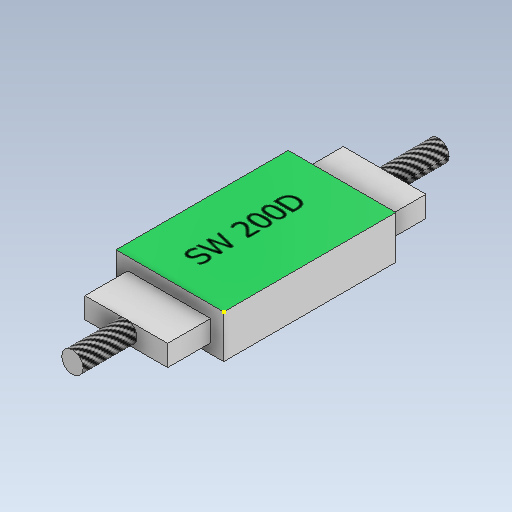
# Autodesk Inventor part: tilt now
Saved by Autodesk Inventor 2021 (Build 250183000, 183)
## iProperties
Created: 2021-07-14
Part Number: tilt now
Material: Generic
Document SubType Name: Modeling
Designer: Dell
Density: 1 g/cm^3
Appearance: Default
Author: Dell
Autodesk Inventor part; units mm, degrees
ref_plane "YZ Plane" through (0, 0, 0) normal (1, 0, 0) x (0, 1, 0)
ref_plane "XZ Plane" through (0, 0, 0) normal (0, 1, 0) x (-1, 0, 0)
ref_plane "XY Plane" through (0, 0, 0) normal (0, 0, 1) x (1, 0, 0)
sketch "Sketch1" plane through (0, 0, 0) normal (0, 1, 0) x (-1, 0, 0)
  line L0 (0, 0) -> (50, 0)
  line L1 (50, 0) -> (50, -80)
  line L2 (50, -80) -> (0, -80)
  line L3 (0, -80) -> (0, 0)
  dimension "d0" = 80
  dimension "d1" = 50
  constraints: 8 end point, 2 parallel, 1 horizontal, 1 perpendicular
  measures "d0" distance of L0.end L1.end
  measures "d1" distance of L1.end L2.end
extrude "Extrusion1" add sketch "Sketch1" along normal blind 20
sketch "Sketch2" plane through (-50, 0, 0) normal (0, 0, 1) x (1, 0, 0)
  line L0 (5.545, 4.5622) -> (43.9524, 4.5622)
  line L1 (43.9524, 4.5622) -> (43.9524, 14.3232)
  line L2 (43.9524, 14.3232) -> (5.545, 14.3232)
  line L3 (5.545, 14.3232) -> (5.545, 4.5622)
  point P0 (50, 0)
  constraints: 8 end point, 2 parallel, 1 horizontal, 1 perpendicular
extrude "Extrusion2" add sketch "Sketch2" along normal blind 20
sketch "Sketch3" plane through (0, 0, -80) normal (0, 0, -1) x (-1, 0, 0)
  line L0 (44.455, 14.3232) -> (6.0476, 14.3232) projected
  line L1 (6.0476, 4.5622) -> (44.455, 4.5622) projected
  line L2 (44.455, 14.3232) -> (6.0476, 14.3232)
  line L3 (6.0476, 14.3232) -> (6.0476, 4.5622)
  line L4 (6.0476, 4.5622) -> (44.455, 4.5622)
  line L5 (44.455, 4.5622) -> (44.455, 14.3232)
  point P0 (0, 0)
  point P1 (6.0476, 14.3232)
  constraints: 8 end point, 2 parallel, 1 horizontal, 1 perpendicular
extrude "Extrusion3" add sketch "Sketch3" along normal blind 20
sketch "Sketch4" plane through (0, 0, -100) normal (0, 0, -1) x (-1, 0, 0)
  circle A0 centre (25.2513, 9.8671) radius 4.9412
  point P0 (0, 0)
  constraints: 1 centre point
extrude "Extrusion4" add sketch "Sketch4" along normal blind 25
sketch "Sketch5" plane through (-50, 0, 20) normal (0, 0, 1) x (1, 0, 0)
  circle A0 centre (24.7487, 9.6549) radius 4.9458
  point P0 (50, 0)
  constraints: 1 centre point
extrude "Extrusion5" add sketch "Sketch5" along normal blind 25
sketch "Sketch6" plane through (0, 20, 0) normal (0, 1, 0) x (1, 0, 0)
  line L0 (-33.19, 13.0471) -> (-33.19, 67.4667) construction
  line L1 (-33.19, 67.4667) -> (-19.8135, 67.4667) construction
  line L2 (-19.8135, 67.4667) -> (-19.8135, 13.0471) construction
  line L3 (-19.8135, 13.0471) -> (-33.19, 13.0471) construction
  point P0 (0, 0)
  constraints: 2 other
body "Solid1"
